L2 (Autodesk Fusion 360 design; units mm, degrees)
part number: 2026-06-01-05-38-21-741
Autodesk Fusion 360 part; units mm, degrees
note: some values were not read from the file. Set by a fixed rule: which face or edge a step refers to.
sketch "Sketch1" plane through (0, 0, 0) normal (0, 0, 1) x (1, 0, 0)
  line L0 (0, 0) -> (100, 0)
  line L1 (100, 0) -> (100, 10)
  line L2 (100, 10) -> (0, 10)
  line L3 (0, 10) -> (0, 0)
  dimension "d1" = 100
  dimension "d2" = 10
  constraint horizontal L0
  constraint vertical L1
  constraint horizontal L2
  constraint vertical L3
  constraint coincident L0.start L3.end
  measures "d1" distance of L0.start L0.end
  measures "d2" distance of L0.start L2.end
extrude "Extrude1" add sketch "Sketch1" along normal blind 10
sketch "Sketch2" plane through (0, 0, 10) normal (0, 0, 1) x (-1, 0, 0)
  line L0 (0, -10) -> (0, 0)
  line L1 (0, 0) -> (-100, 0)
  line L2 (-100, 0) -> (-100, -10)
  line L3 (-100, -10) -> (0, -10)
  circle A0 centre (-5, -5) radius 4.5
  circle A1 centre (-25, -5) radius 4.5
  circle A2 centre (-45, -5) radius 4.5
  circle A3 centre (-65, -5) radius 4.5
  circle A4 centre (-85, -5) radius 4.5
  dimension "d5" = 9
  dimension "d6" = 9
  dimension "d7" = 9
  dimension "d8" = 9
  dimension "d9" = 9
  measures "d5" diameter of A0
  measures "d6" diameter of A1
  measures "d7" diameter of A2
  measures "d8" diameter of A3
  measures "d9" diameter of A4
extrude "Extrude2" cut sketch "Sketch2" against normal blind 20 contours A0 | A1 | A2 | A3 | A4
sketch "Sketch3" plane through (0, 0, 0) normal (0, -1, 0) x (1, 0, 0)
  line L0 (0, 0) -> (100, 0)
  line L1 (100, 0) -> (100, 10)
  line L2 (100, 10) -> (0, 10)
  line L3 (0, 10) -> (0, 0)
  circle A0 centre (75, 5) radius 4.5
  circle A1 centre (55, 5) radius 4.5
  circle A2 centre (35, 5) radius 4.5
  circle A3 centre (15, 5) radius 4.5
  dimension "d12" = 9
  dimension "d13" = 9
  dimension "d14" = 9
  dimension "d15" = 9
  measures "d12" diameter of A0
  measures "d13" diameter of A1
  measures "d14" diameter of A2
  measures "d15" diameter of A3
extrude "Extrude3" cut sketch "Sketch3" against normal blind 10 contours A0 | A1 | A2 | A3
sketch "Sketch4" plane through (100, 0, 0) normal (1, 0, 0) x (0, 1, 0)
  line L0 (0, 0) -> (10, 0)
  line L1 (10, 0) -> (10, 10)
  line L2 (10, 10) -> (0, 10)
  line L3 (0, 10) -> (0, 0)
  circle A0 centre (5, 5) radius 4
  dimension "d18" = 8
  measures "d18" diameter of A0
extrude "Extrude4" cut sketch "Sketch4" against normal blind 3 contours A0
sketch "Sketch5" plane through (0, 0, 0) normal (1, 0, 0) x (0, 1, 0)
  circle A0 centre (5, 5) radius 4
  circle A1 centre (5, 5) radius 3.5
  dimension "d21" = 8
  dimension "d22" = 7
  constraint concentric A0 A1
  measures "d21" diameter of A0
  measures "d22" diameter of A1
extrude "Extrude5" add sketch "Sketch5" against normal blind 3
extrude "Extrude6" add 1 faces at (-3, 8.8054, 4.6274) along direction (1, 0, 0) blind 3
extrude "Extrude7" add 1 faces at (-3, 8.8054, 4.6274) along direction (1, 0, 0) blind 3
extrude "Extrude8" cut 1 faces at (-3, 8.8054, 4.6274) along direction (1, 0, 0) blind 3.5
extrude "Extrude9" add 2 faces at (0.5, 5.3558, 8.8079) (0.5, 4.8013, 1.1816) along direction (-1, 0, 0) blind 0.5
sketch "Sketch6" plane through (0, 0, 0) normal (-1, 0, 0) x (0, -1, 0)
  line L0 (-10, 0) -> (0, 0)
  line L1 (0, 0) -> (0, 10)
  line L2 (0, 10) -> (-10, 10)
  line L3 (-10, 10) -> (-10, 0)
  circle A0 centre (-5, 5) radius 4.5
  circle A1 centre (-5, 5) radius 4
  dimension "d33" = 9
  dimension "d34" = 8
  constraint concentric A0 A1
  measures "d33" diameter of A0
  measures "d34" diameter of A1
sketch "Sketch7" plane through (0, 0, 0) normal (-1, 0, 0) x (0, -1, 0)
extrude "Extrude10" add sketch "Sketch6" along normal blind 3 contours A0
